Autodesk Fusion 360 part; units mm, degrees
(part 4 of 4)
extrude "Extrude42" cut 1 faces at (241.9748, -67.9493, 0.1667) along direction (0.70694, 0.707274, 0) blind 0.1 on bodies 2 bodies 2
extrude "Extrude43" cut 3 faces at (-100.9455, 8.4316, 1.9) (-86.8033, 22.3527, 1.9) (-74.7903, 37.7926, 1.9) along direction (0, 0, -1) blind 1.4 on bodies 1 bodies 1
extrude "Extrude44" add sketch "Sketch30" along normal blind 2 contours A11 A44 | A11 A44 | A11 A42 | A11 A42 | A40 | A46 bodies 1
sphere "SpherePrimitive29" add diameter 5 placed x (-1, 0, 0) y (0, -1, 0) z (0, 0, 1) at (-112.9992, 6.508, 2.5) bodies 1
sphere "SpherePrimitive30" add diameter 5 placed x (-1, 0, 0) y (0, -1, 0) z (0, 0, 1) at (-105.9992, 6.508, 2.5) bodies 1
sphere "SpherePrimitive31" add diameter 5 placed x (-1, 0, 0) y (0, -1, 0) z (0, 0, 1) at (-98.9994, 6.5337, 2.5) bodies 1
sphere "SpherePrimitive32" add diameter 5 placed x (-1, 0, 0) y (0, -1, 0) z (0, 0, 1) at (-92, 6.508, 2.5) bodies 1
extrude "Extrude45" cut sketch "Sketch30" along normal blind 2 contours L30 A48 | L30 A48 | A11 A44 A50 | A11 A44 A50 | A11 A42 A49 | A11 A42 A49 | A51 bodies 1
extrude "Extrude46" add sketch "Sketch38" against normal blind 0.5 contours A36 L124 | A97 | A36 L90 L110 L112 L114 A95 L122 L124 | L88 L89 L90 L114 L123 L124 | L112 A95 | A81 | A83 | A85 | A87 | A89 | A91 | A93 | L92 A95 L120 L121 L122 L124 L125 | L88 L123 L126 | L92 A95 | A71 A72 | A79 | A77 | A75 | A73 picked at (-177.0875, 13.79) picked at (-237.4452, 8.1088) bodies 2 makes body 3 at (268, -8.492, 0)
extrude "Extrude47" add sketch "Sketch38" against normal blind 0.5 contours L92 L112 A95 L124 | L92 L112 A95 | L92 L112 A95 L122 bodies 2 3
extrude "Extrude48" cut sketch "Sketch38" against normal blind 2 contours L92 L105 L108 L111 | A59 | A57 | A55 | A53 | A51 | A49 | A47 | A45 | A43 | L92 L93 L105 L106 L107 L108 | A61 A62 | A69 | A67 | A65 | A63 picked at (-237.4452, -6.8912) bodies 2
sketch "Sketch43" plane through (0, 0, 0.5) normal (0, 0, 1) x (-1, 0, 0)
  line L0 (-170, 0) -> (-170, -62.2885)
  line L1 (-170, -62.2885) -> (-270, -62.2885)
  line L2 (-270, -62.2885) -> (-270, -75)
  line L3 (-270, -75) -> (-170, -75)
  line L4 (-170, -75) -> (-170, -80)
  line L5 (-170, -80) -> (-102.5, -80)
  line L6 (-102.5, -80) -> (-80, -75)
  line L7 (-80, -75) -> (-10, -75)
  line L8 (-10, -75) -> (-10, -61.9841)
  line L9 (-10, -61.9841) -> (-80, -61.9841)
  line L10 (-80, -61.9841) -> (-80, -13.016)
  line L11 (-80, -13.016) -> (-10, -13.016)
  line L12 (-10, -13.016) -> (-10, 0)
  line L13 (-10, 0) -> (-80, 0)
  line L14 (-80, 0) -> (-108.0327, 6.2295)
  line L15 (-108.0327, 6.2295) -> (-123.7944, 15)
  line L16 (-123.7944, 15) -> (-270, 15)
  line L17 (-270, 15) -> (-270, 1.984)
  line L18 (-270, 1.984) -> (-167.1743, 1.984)
  line L19 (-167.1743, 1.984) -> (-170, 0)
  circle A0 centre (-262.5, 8.492) radius 1.5
  circle A1 centre (-255.5, 8.492) radius 1.5
  circle A2 centre (-213.5, 8.492) radius 1.5
  circle A3 centre (-206.5, 8.492) radius 1.5
  circle A4 centre (-199.5, 8.492) radius 1.5
  circle A5 centre (-234.5, 8.492) radius 1.5
  circle A6 centre (-192.5, 8.492) radius 1.5
  circle A7 centre (-220.5, 8.492) radius 1.5
  circle A8 centre (-248.5, 8.492) radius 1.5
  circle A9 centre (-227.5, 8.492) radius 1.5
  circle A10 centre (-241.5, 8.492) radius 1.5
  circle A11 centre (-185.5, 8.492) radius 1.5
  circle A12 centre (-171.5, 8.492) radius 1.5
  circle A13 centre (-178.5, 8.492) radius 1.5
  line L20 (-154.2321, 4.5244) -> (-127.1667, 4.5244)
  line L21 (-127.1667, 4.5244) -> (-122.1059, 3.6443)
  arc A14 (-157.8415, -38.9188) -> (-122.1059, 3.6443) centre (-208.4491, 39.8542) ccw
  line L22 (-157.8415, -38.9188) -> (-157.8415, -35.4188)
  line L23 (-157.8415, -35.4188) -> (-161.6623, -35.4188)
  line L24 (-161.6623, -35.4188) -> (-161.6623, 0)
  line L25 (-161.6623, 0) -> (-154.2321, 4.5244)
  line L26 (-125, -57) -> (-85, -57)
  line L27 (-85, -57) -> (-85, -60)
  line L28 (-85, -60) -> (-125, -60)
  arc A15 (-125, -60) -> (-146.3234, -75) centre (-125, -82.6562) ccw
  line L29 (-146.3234, -75) -> (-149.4872, -75)
  arc A16 (-125, -57) -> (-149.4872, -75) centre (-125, -82.6562) ccw
  line L30 (-139.25, -71.5367) -> (-133.25, -71.5367)
  line L31 (-133.25, -71.5367) -> (-133.25, -74.5367)
  line L32 (-133.25, -74.5367) -> (-139.25, -74.5367)
  line L33 (-139.25, -74.5367) -> (-139.25, -71.5367)
  line L34 (-106.6893, -51.989) -> (-112.6017, -50.9672)
  line L35 (-112.6017, -50.9672) -> (-112.0908, -48.011)
  line L36 (-112.0908, -48.011) -> (-106.1784, -49.0328)
  line L37 (-106.1784, -49.0328) -> (-106.6893, -51.989)
  line L38 (-108.0908, -25.011) -> (-102.1784, -26.0328)
  line L39 (-102.1784, -26.0328) -> (-102.6893, -28.989)
  line L40 (-102.6893, -28.989) -> (-108.6017, -27.9672)
  line L41 (-108.6017, -27.9672) -> (-108.0908, -25.011)
  line L42 (-115.0324, 0.9507) -> (-109.0325, 0.9195)
  line L43 (-109.0325, 0.9195) -> (-109.0481, -2.0804)
  line L44 (-109.0481, -2.0804) -> (-115.048, -2.0492)
  line L45 (-115.048, -2.0492) -> (-115.0324, 0.9507)
  line L46 (-104.686, 0.859) -> (-98.6861, 0.8794)
  line L47 (-98.6861, 0.8794) -> (-98.6759, -2.1206)
  line L48 (-98.6759, -2.1206) -> (-104.6759, -2.141)
  line L49 (-104.6759, -2.141) -> (-104.686, 0.859)
  line L50 (-123.7607, -25.5524) -> (-118.1333, -27.6339)
  line L51 (-118.1333, -27.6339) -> (-119.174, -30.4476)
  line L52 (-119.174, -30.4476) -> (-124.8014, -28.3661)
  line L53 (-124.8014, -28.3661) -> (-123.7607, -25.5524)
  line L54 (-130.7607, -47.5524) -> (-125.1333, -49.6339)
  line L55 (-125.1333, -49.6339) -> (-126.174, -52.4476)
  line L56 (-126.174, -52.4476) -> (-131.8014, -50.3661)
  line L57 (-131.8014, -50.3661) -> (-130.7607, -47.5524)
  line L58 (-116.75, -71.5367) -> (-110.75, -71.5367)
  line L59 (-110.75, -71.5367) -> (-110.75, -74.5367)
  line L60 (-110.75, -74.5367) -> (-116.75, -74.5367)
  line L61 (-116.75, -74.5367) -> (-116.75, -71.5367)
  line L62 (-161.75, -71.5367) -> (-155.75, -71.5367)
  line L63 (-155.75, -71.5367) -> (-155.75, -74.5367)
  line L64 (-155.75, -74.5367) -> (-161.75, -74.5367)
  line L65 (-161.75, -74.5367) -> (-161.75, -71.5367)
  line L66 (-91.9719, -47.9791) -> (-86.0721, -49.071)
  line L67 (-86.0721, -49.071) -> (-86.6181, -52.0209)
  line L68 (-86.6181, -52.0209) -> (-92.5179, -50.929)
  line L69 (-92.5179, -50.929) -> (-91.9719, -47.9791)
  line L70 (-90.5728, -25.1023) -> (-84.573, -25.1532)
  line L71 (-84.573, -25.1532) -> (-84.5984, -28.1531)
  line L72 (-84.5984, -28.1531) -> (-90.5982, -28.1022)
  line L73 (-90.5982, -28.1022) -> (-90.5728, -25.1023)
  line L74 (-122.179, 1.1199) -> (-116.1792, 1.0739)
  line L75 (-116.1792, 1.0739) -> (-116.2025, -1.9678)
  line L76 (-116.2025, -1.9678) -> (-122.2023, -1.9219)
  line L77 (-122.2023, -1.9219) -> (-122.179, 1.1199)
  line L78 (-90.5728, -3.1023) -> (-84.573, -3.1532)
  line L79 (-84.573, -3.1532) -> (-84.5984, -6.1531)
  line L80 (-84.5984, -6.1531) -> (-90.5982, -6.1022)
  line L81 (-90.5982, -6.1022) -> (-90.5728, -3.1023)
  line L82 (-138.1594, -27.0213) -> (-133.271, -30.5004)
  line L83 (-133.271, -30.5004) -> (-135.0348, -32.9787)
  line L84 (-135.0348, -32.9787) -> (-139.9232, -29.4996)
  line L85 (-139.9232, -29.4996) -> (-138.1594, -27.0213)
  line L86 (-152.1594, -47.0213) -> (-147.271, -50.5004)
  line L87 (-147.271, -50.5004) -> (-149.0348, -52.9787)
  line L88 (-149.0348, -52.9787) -> (-153.9232, -49.4996)
  line L89 (-153.9232, -49.4996) -> (-152.1594, -47.0213)
  line L90 (-94.25, -68.5) -> (-88.25, -68.5)
  line L91 (-88.25, -68.5) -> (-88.25, -71.5)
  line L92 (-88.25, -71.5) -> (-94.25, -71.5)
  line L93 (-94.25, -71.5) -> (-94.25, -68.5)
  circle A17 centre (-249, -68.6442) radius 1.5
  circle A18 centre (-221, -68.6442) radius 1.5
  circle A19 centre (-193, -68.6442) radius 1.5
  circle A20 centre (-214, -68.6442) radius 1.5
  circle A21 centre (-242, -68.6442) radius 1.5
  circle A22 centre (-256, -68.6442) radius 1.5
  circle A23 centre (-228, -68.6442) radius 1.5
  circle A24 centre (-200, -68.6442) radius 1.5
  circle A25 centre (-207, -68.6442) radius 1.5
  circle A26 centre (-235, -68.6442) radius 1.5
  circle A27 centre (-263, -68.6442) radius 1.5
  line L94 (-129.2268, -20.3093) -> (-121.9977, -4.5677)
  line L95 (-121.9977, -4.5677) -> (-97.7598, -4.7733)
  line L96 (-97.7598, -4.7733) -> (-85, -9.2623)
  line L97 (-85, -9.2623) -> (-85.0969, -20.6836)
  line L98 (-85.0969, -20.6836) -> (-129.2268, -20.3093)
  line L99 (-85, -35.2698) -> (-85.0893, -45.8041)
  line L100 (-85.0893, -45.8041) -> (-159.6826, -45.1714)
  line L101 (-159.6826, -45.1714) -> (-144.4557, -34.7655)
  line L102 (-144.4557, -34.7655) -> (-85, -35.2698)
  line L103 (-144.4557, -59.7611) -> (-150.6729, -68.3891)
  line L104 (-150.6729, -68.3891) -> (-167.8309, -68.3891)
  line L105 (-167.8309, -68.3891) -> (-167.8309, -48.5956)
  line L106 (-167.8309, -48.5956) -> (-144.4557, -59.7611)
  circle A28 centre (-172, -68.6442) radius 1.5
  circle A29 centre (-179, -68.6442) radius 1.5
  circle A30 centre (-186, -68.6442) radius 1.5
  circle A31 centre (-46.5, -68.4921) radius 1.5
  circle A32 centre (-53.5, -68.4921) radius 1.5
  circle A33 centre (-32.5, -68.4921) radius 1.5
  circle A34 centre (-25.5, -68.4921) radius 1.5
  circle A35 centre (-18.5, -68.4921) radius 1.5
  circle A36 centre (-67.5, -68.4921) radius 1.5
  circle A37 centre (-60.5, -68.4921) radius 1.5
  circle A38 centre (-39.5, -68.4921) radius 1.5
  circle A39 centre (-39.5, -6.508) radius 1.5
  circle A40 centre (-46.5, -6.508) radius 1.5
  circle A41 centre (-74.5, -6.508) radius 1.5
  circle A42 centre (-67.5, -6.508) radius 1.5
  circle A43 centre (-60.5, -6.508) radius 1.5
  circle A44 centre (-18.5, -6.508) radius 1.5
  circle A45 centre (-25.5, -6.508) radius 1.5
  circle A46 centre (-53.5, -6.508) radius 1.5
  circle A47 centre (-32.5, -6.508) radius 1.5
  line L107 (-157.8415, -38.9188) -> (-170, -41.622)
  line L108 (-170, -41.622) -> (-170, 0)
  line L109 (-170, 0) -> (-167.1743, 1.984)
  line L110 (-167.1743, 1.984) -> (-154.2321, 4.5244)
  line L111 (-154.2321, 4.5244) -> (-161.6623, 0)
  line L112 (-161.6623, 0) -> (-161.6623, -35.4188)
  line L113 (-161.6623, -35.4188) -> (-157.8415, -35.4188)
  line L114 (-157.8415, -35.4188) -> (-157.8415, -38.9188)
  constraint coincident A14.start L22.start
  constraint coincident L0 L107.end
  constraint coincident L0.start L19.end
  constraint parallel L0 L108
  constraint coincident L18.end L19.start
  constraint coincident L20.start L25.end
  constraint coincident L24.end L25.start
  constraint coincident L23.end L24.start
  constraint coincident L22.end L23.start
extrude "Extrude49" cut sketch "Sketch43" against normal blind 5 contours L0 L19 L22 L23 L24 L25 L107 L108 L109 L110 L111 L112 L113 L114 bodies 2
extrude "Extrude50" cut 1 faces at (270, -6.3227, 0.3333) along direction (-1, 0, 0) blind 65 on bodies 2 bodies 2
delete_face "DeleteFace11" 2 faces at (171.3157, 67.3094, 0.3333) (178.3157, 67.3094, 0.3333) on bodies 2
extrude "Extrude51" cut 1 faces at (270, 66.5257, 0.1667) along direction (-1, 0, 0) blind 58 on bodies 2 bodies 2
extrude "Extrude52" cut 1 faces at (10, 70.6614, 0.3333) along direction (1, 0, 0) blind 31 on bodies 2 bodies 2
extrude "Extrude53" cut 1 faces at (10, 4.3387, 0.3333) along direction (1, 0, 0) blind 40 on bodies 2 bodies 2
delete_face "DeleteFace12" 6 faces at (-68.6882, 70.4935, 1.1667) (-75.6882, 70.4935, 1.1667) (-82.6882, 70.4935, 1.1667) (-78.2714, 70, 2.8263) (-71.2714, 70, 2.8263) (-64.2714, 70, 2.8263) on bodies 1
delete_face "DeleteFace13" 4 faces at (-75.6766, 5.0084, 1.1667) (-68.6766, 5.0084, 1.1667) (-67.5214, 6.508, 2.8263) (-74.5214, 6.508, 2.8263) on bodies 1
